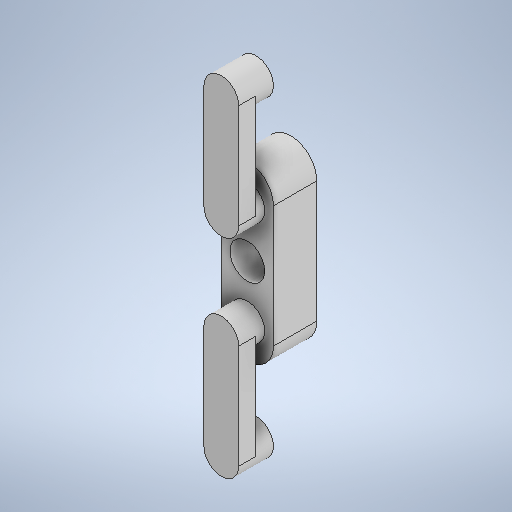
# Autodesk Inventor part: Button Cap
Saved by Autodesk Inventor 2026 (Build 300175050, 175E)
## iProperties
Created: 2025-07-10
Part Number: Button Cap
Material: Generic
Document SubType Name: Modeling
Designer: Jochen Alt
Density: 1 g/cm^3
Appearance: Default
Author: Jochen Alt
Autodesk Inventor part; units mm, degrees
ref_plane "YZ Plane" through (0, 0, 0) normal (1, 0, 0) x (0, 1, 0)
ref_plane "XZ Plane" through (0, 0, 0) normal (0, 1, 0) x (-1, 0, 0)
ref_plane "XY Plane" through (0, 0, 0) normal (0, 0, 1) x (1, 0, 0)
sketch "Sketch1" plane through (0, 0, 0) normal (0, 0, 1) x (1, 0, 0)
  line L0 (-2.1, 0) -> (2.1, 0) construction
  line L1 (0, 14) -> (0, -14) construction
  line L2 (0, 3.5) -> (0, -3.5) construction
  line L3 (-1.5, 3.5) -> (-1.5, -3.5)
  line L4 (1.5, -3.5) -> (1.5, 3.5)
  arc A0 (1.5, 3.5) -> (-1.5, 3.5) centre (0, 3.5) ccw
  arc A1 (-1.5, -3.5) -> (1.5, -3.5) centre (0, -3.5) ccw
  circle A2 centre (0, 0) radius 1
  line L5 (-1, 4.618) -> (-1, 9)
  arc A3 (1, 9) -> (-1, 9) centre (0, 9) ccw
  line L6 (1, 9) -> (1, 4.618)
  line L7 (-1, 4.618) -> (-1, 3)
  arc A4 (-1, 3) -> (1, 3) centre (0, 3) ccw
  line L8 (1, 4.618) -> (1, 3)
  arc A5 (1, 3) -> (-1, 3) centre (0, 3) ccw
  arc A6 (-1, 9) -> (1, 9) centre (0, 9) ccw
  line L9 (-1, -4.618) -> (-1, -9)
  arc A7 (-1, -9) -> (1, -9) centre (0, -9) ccw
  line L10 (1, -9) -> (1, -4.618)
  line L11 (-1, -4.618) -> (-1, -3)
  arc A8 (1, -3) -> (-1, -3) centre (0, -3) ccw
  line L12 (1, -4.618) -> (1, -3)
  arc A9 (-1, -3) -> (1, -3) centre (0, -3) ccw
  arc A10 (1, -9) -> (-1, -9) centre (0, -9) ccw
  dimension "d0" = 1.5
  dimension "d1" = 7
  dimension "d2" = 2
  dimension "d7" = 3
  dimension "d8" = 1
  dimension "d9" = 6
  constraints: 24 end point, 22 point on circle, 11 centre point, 11 symmetric about line, 9 tangent, 4 point on line, 4 vertical, 2 coincident, 2 equal radius, 1 midpoint, 1 parallel, 5 other
  measures "d0" radius of A0
  measures "d1" distance of L4.start L4.end
  measures "d2" diameter of A2
  measures "d7" distance of point (0, 0) A4.centre
  measures "d8" radius of A4
  measures "d9" distance of A5.centre A3.centre
extrude "Extrusion1" add sketch "Sketch1" along normal blind 1 contours A0 L7 A4 L8 L4 A1 L12 A8 L11 L3 | A0 L8 A5 L7 | L11 A9 L12 A1 | A5 A4 | A8 A9 | A2
extrude "Extrusion2" add sketch "Sketch1" along normal blind 1.5 from surface at 1 contours A0 L7 A4 L8 L4 A1 L12 A8 L11 L3 | A0 L8 A5 L7 | L11 A9 L12 A1 | A5 A4 | A8 A9
extrude "Extrusion3" add sketch "Sketch1" along normal blind 0.5 from surface at 2.5 contours A5 A4 | A8 A9
extrude "Extrusion4" add sketch "Sketch1" along normal blind 1 from surface at 3 contours L5 A6 L6 A0 | A0 L8 A5 L7 | L11 A9 L12 A1 | A1 L10 A10 L9 | A3 A6 | A5 A4 | A10 A7 | A8 A9
extrude "Extrusion5" add sketch "Sketch1" against normal blind 1 from surface at 3 contours A3 A6 | A10 A7
body "Solid1"
